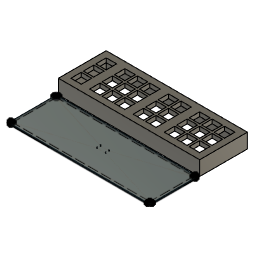
TIX Clock v4 (Autodesk Fusion 360 design; units mm, degrees)
Autodesk Fusion 360 part; units mm, degrees
note: some values were not read from the file. Set by a fixed rule: which face or edge a step refers to.
sketch "Sketch3" plane through (0, 0, 0) normal (0, 0, 1) x (1, 0, 0)
  line L0 (0, 0) -> (680, 0)
  line L1 (680, 0) -> (680, 230)
  line L2 (680, 230) -> (0, 230)
  line L3 (0, 230) -> (0, 0)
  dimension "d16" = 680
  dimension "d17" = 230
  constraint horizontal L0
  constraint vertical L1
  constraint horizontal L2
  constraint vertical L3
  constraint coincident L0.start L3.end
  measures "d16" distance of L0.start L0.end
  measures "d17" distance of L0.start L2.end
extrude "Extrude1" add sketch "Sketch3" along normal blind 70 makes body 1
sketch "Sketch4" plane through (0, 0, 70) normal (0, 0, 1) x (-1, 0, 0)
  line L0 (0, -230) -> (0, 0) construction
  line L1 (0, 0) -> (-680, 0)
  line L2 (-680, 0) -> (-680, -230)
  line L3 (-680, -230) -> (0, -230)
  line L4 (0, -200) -> (-680, -200)
  line L5 (0, -30) -> (-680, -30)
  line L6 (-30, -230) -> (-30, 0)
  line L7 (-650, -230) -> (-650, 0)
  line L8 (-80, -200) -> (-80, -30)
  line L9 (-120, -200) -> (-120, -30)
  line L10 (-170, -200) -> (-170, -30)
  line L11 (-180, -200) -> (-180, -30)
  line L12 (-230, -200) -> (-230, -30)
  line L13 (-30, -150) -> (-650, -150)
  line L14 (-30, -140) -> (-650, -140)
  line L15 (-30, -90) -> (-650, -90)
  line L16 (-30, -80) -> (-650, -80)
  line L17 (-30, -30) -> (-650, -30)
  line L18 (-240, -200) -> (-240, -30)
  line L19 (-290, -200) -> (-290, -30)
  line L20 (-330, -200) -> (-330, -30)
  line L21 (-380, -200) -> (-380, -30)
  line L22 (-390, -200) -> (-390, -30)
  line L23 (-440, -200) -> (-440, -30)
  line L24 (-480, -200) -> (-480, -30)
  line L25 (-530, -200) -> (-530, -30)
  line L26 (-540, -200) -> (-540, -30)
  line L27 (-590, -200) -> (-590, -30)
  line L28 (-600, -200) -> (-600, -30)
  line L29 (-650, -200) -> (-650, -30) construction
  dimension "d21" = 30
  dimension "d22" = 30
  dimension "d23" = 30
  dimension "d24" = 30
  dimension "d25" = 50
  dimension "d26" = 40
  dimension "d27" = 50
  dimension "d28" = 10
  dimension "d29" = 50
  dimension "d30" = 50
  dimension "d31" = 10
  dimension "d32" = 50
  dimension "d33" = 10
  dimension "d34" = 50
  dimension "d35" = 10
  dimension "d36" = 50
  dimension "d37" = 40
  dimension "d38" = 50
  dimension "d39" = 10
  dimension "d40" = 50
  dimension "d41" = 40
  dimension "d42" = 50
  dimension "d43" = 10
  dimension "d44" = 50
  dimension "d45" = 10
  dimension "d46" = 50
  constraint coincident L0 L4.start
  constraint perpendicular L0 L4
  constraint coincident L2 L4.end
  constraint coincident L0 L5.start
  constraint coincident L2 L5.end
  constraint perpendicular L2 L5
  constraint coincident L3 L6.start
  constraint coincident L1 L6.end
  constraint perpendicular L1 L6
  constraint coincident L3 L7.start
  constraint coincident L1 L7.end
  constraint perpendicular L1 L7
  constraint coincident L4 L8.start
  constraint coincident L5 L8.end
  constraint perpendicular L5 L8
  constraint coincident L4 L9.start
  constraint coincident L5 L9.end
  constraint perpendicular L5 L9
  constraint coincident L4 L10.start
  constraint coincident L5 L10.end
  constraint perpendicular L5 L10
  constraint coincident L4 L11.start
  constraint coincident L5 L11.end
  constraint perpendicular L5 L11
  constraint coincident L4 L12.start
  constraint coincident L5 L12.end
  constraint perpendicular L5 L12
  constraint coincident L7 L13.end
  constraint perpendicular L7 L13
  constraint coincident L6 L14.start
  constraint coincident L7 L14.end
  constraint perpendicular L7 L14
  constraint coincident L6 L15.start
  constraint coincident L7 L15.end
  constraint perpendicular L7 L15
  constraint coincident L6 L16.start
  constraint coincident L7 L16.end
  constraint perpendicular L7 L16
  constraint coincident L6 L17.start
  constraint coincident L7 L17.end
  constraint perpendicular L7 L17
  constraint coincident L4 L18.start
  constraint coincident L5 L18.end
  constraint coincident L4 L19.start
  constraint coincident L17 L19.end
  constraint coincident L4 L20.start
  constraint perpendicular L4 L20
  constraint coincident L4 L21.start
  constraint coincident L5 L21.end
  constraint coincident L4 L22.start
  constraint coincident L17 L22.end
  constraint coincident L4 L23.start
  constraint coincident L5 L23.end
  constraint perpendicular L5 L23
  constraint perpendicular L13 L24
  constraint coincident L4 L25.start
  constraint coincident L5 L25.end
  constraint coincident L4 L26.start
  constraint coincident L5 L26.end
  constraint coincident L4 L27.start
  constraint coincident L17 L27.end
  constraint coincident L4 L28.start
  constraint coincident L5 L28.end
  constraint coincident L4 L29.start
  constraint coincident L5 L17.end
  measures "d21" distance of L3 L4
  measures "d22" distance of L1 L5
  measures "d23" distance of L0 L6
  measures "d24" distance of L2 L7
  measures "d25" distance of L6 L8
  measures "d26" distance of L8 L9
  measures "d27" distance of L9 L10
  measures "d28" distance of L10 L11
  measures "d29" distance of L11 L12
  measures "d30" distance of L4 L13
  measures "d31" distance of L13 L14
  measures "d32" distance of L14 L15
  measures "d33" distance of L15 L16
  measures "d34" distance of L16 L17
  measures "d35" distance of L12 L18
  measures "d36" distance of L18 L19
  measures "d37" distance of L19 L20
  measures "d38" distance of L20 L21
  measures "d39" distance of L21 L22
  measures "d40" distance of L22 L23
  measures "d41" distance of L23 L24
  measures "d42" distance of L24 L25
  measures "d43" distance of L25 L26
  measures "d44" distance of L26 L27
  measures "d45" distance of L27 L28
  measures "d46" distance of L28 L29
extrude "Extrude2" cut sketch "Sketch4" against normal blind 170 contours L5 L6 L8 L16 L17 | L5 L7 L16 L17 L28 | L5 L9 L10 L16 L17 | L6 L8 L14 L15 | L5 L16 L17 L26 L27 | L7 L14 L15 L28 | L4 L7 L13 L28 | L5 L11 L12 L16 L17 | L9 L10 L14 L15 | L4 L6 L8 L13 | L5 L16 L17 L24 L25 | L14 L15 L26 L27 | L4 L13 L26 L27 | L5 L16 L17 L18 L19 | L11 L12 L14 L15 | L4 L9 L10 L13 | L5 L16 L17 L22 L23 | L14 L15 L24 L25 | L4 L13 L24 L25 | L5 L16 L17 L20 L21 | L14 L15 L18 L19 | L4 L11 L12 L13 | L14 L15 L22 L23 | L4 L13 L22 L23 | L14 L15 L20 L21 | L4 L13 L18 L19 | L4 L13 L20 L21 bodies 1
sketch "Sketch5" plane through (0, 0, 0) normal (0, 0, -1) x (1, 0, 0)
  line L0 (650, -30) -> (650, -80)
  line L1 (650, -80) -> (600, -80)
  line L2 (600, -80) -> (600, -30)
  line L3 (600, -30) -> (650, -30)
  line L4 (480, -150) -> (530, -150)
  line L5 (530, -150) -> (530, -200)
  line L6 (530, -200) -> (480, -200)
  line L7 (480, -200) -> (480, -150)
  line L8 (440, -90) -> (440, -140)
  line L9 (440, -140) -> (390, -140)
  line L10 (390, -140) -> (390, -90)
  line L11 (390, -90) -> (440, -90)
  line L12 (380, -30) -> (380, -80)
  line L13 (380, -80) -> (330, -80)
  line L14 (330, -80) -> (330, -30)
  line L15 (330, -30) -> (380, -30)
  line L16 (180, -200) -> (180, -150)
  line L17 (180, -150) -> (230, -150)
  line L18 (230, -150) -> (230, -200)
  line L19 (230, -200) -> (180, -200)
  line L20 (120, -140) -> (120, -90)
  line L21 (120, -90) -> (170, -90)
  line L22 (170, -90) -> (170, -140)
  line L23 (170, -140) -> (120, -140)
  line L24 (30, -30) -> (80, -30)
  line L25 (80, -30) -> (80, -80)
  line L26 (80, -80) -> (30, -80)
  line L27 (30, -80) -> (30, -30)
  line L28 (120, -200) -> (120, -150)
  line L29 (120, -150) -> (170, -150)
  line L30 (170, -150) -> (170, -200)
  line L31 (170, -200) -> (120, -200)
  line L32 (180, -140) -> (180, -90)
  line L33 (180, -90) -> (230, -90)
  line L34 (230, -90) -> (230, -140)
  line L35 (230, -140) -> (180, -140)
  line L36 (290, -30) -> (290, -80)
  line L37 (290, -80) -> (240, -80)
  line L38 (240, -80) -> (240, -30)
  line L39 (240, -30) -> (290, -30)
  line L40 (390, -150) -> (440, -150)
  line L41 (440, -150) -> (440, -200)
  line L42 (440, -200) -> (390, -200)
  line L43 (390, -200) -> (390, -150)
  line L44 (530, -90) -> (530, -140)
  line L45 (530, -140) -> (480, -140)
  line L46 (480, -140) -> (480, -90)
  line L47 (480, -90) -> (530, -90)
  line L48 (590, -30) -> (590, -80)
  line L49 (590, -80) -> (540, -80)
  line L50 (540, -80) -> (540, -30)
  line L51 (540, -30) -> (590, -30)
  line L52 (650, -90) -> (650, -140)
  line L53 (650, -140) -> (600, -140)
  line L54 (600, -140) -> (600, -90)
  line L55 (600, -90) -> (650, -90)
  line L56 (540, -150) -> (590, -150)
  line L57 (590, -150) -> (590, -200)
  line L58 (590, -200) -> (540, -200)
  line L59 (540, -200) -> (540, -150)
  line L60 (440, -30) -> (440, -80)
  line L61 (440, -80) -> (390, -80)
  line L62 (390, -80) -> (390, -30)
  line L63 (390, -30) -> (440, -30)
  line L64 (380, -90) -> (380, -140)
  line L65 (380, -140) -> (330, -140)
  line L66 (330, -140) -> (330, -90)
  line L67 (330, -90) -> (380, -90)
  line L68 (240, -150) -> (290, -150)
  line L69 (290, -150) -> (290, -200)
  line L70 (290, -200) -> (240, -200)
  line L71 (240, -200) -> (240, -150)
  line L72 (120, -80) -> (120, -30)
  line L73 (120, -30) -> (170, -30)
  line L74 (170, -30) -> (170, -80)
  line L75 (170, -80) -> (120, -80)
  line L76 (30, -90) -> (80, -90)
  line L77 (80, -90) -> (80, -140)
  line L78 (80, -140) -> (30, -140)
  line L79 (30, -140) -> (30, -90)
  line L80 (30, -150) -> (80, -150)
  line L81 (80, -150) -> (80, -200)
  line L82 (80, -200) -> (30, -200)
  line L83 (30, -200) -> (30, -150)
  line L84 (180, -80) -> (180, -30)
  line L85 (180, -30) -> (230, -30)
  line L86 (230, -30) -> (230, -80)
  line L87 (230, -80) -> (180, -80)
  line L88 (290, -90) -> (290, -140)
  line L89 (290, -140) -> (240, -140)
  line L90 (240, -140) -> (240, -90)
  line L91 (240, -90) -> (290, -90)
  line L92 (330, -150) -> (380, -150)
  line L93 (380, -150) -> (380, -200)
  line L94 (380, -200) -> (330, -200)
  line L95 (330, -200) -> (330, -150)
  line L96 (530, -30) -> (530, -80)
  line L97 (530, -80) -> (480, -80)
  line L98 (480, -80) -> (480, -30)
  line L99 (480, -30) -> (530, -30)
  line L100 (590, -90) -> (590, -140)
  line L101 (590, -140) -> (540, -140)
  line L102 (540, -140) -> (540, -90)
  line L103 (540, -90) -> (590, -90)
  line L104 (600, -200) -> (600, -150)
  line L105 (600, -150) -> (650, -150)
  line L106 (650, -150) -> (650, -200)
  line L107 (650, -200) -> (600, -200)
  line L108 (0, 0) -> (0, -230)
  line L109 (0, -230) -> (680, -230)
  line L110 (680, -230) -> (680, 0)
  line L111 (680, 0) -> (0, 0)
  line L112 (20, 0) -> (20, -230)
  line L113 (0, -20) -> (680, -20)
  line L114 (660, 0) -> (660, -230)
  line L115 (680, -210) -> (0, -210)
  dimension "d50" = 20
  dimension "d51" = 20
  dimension "d52" = 20
  dimension "d53" = 20
  constraint coincident L111 L112.start
  constraint coincident L109 L112.end
  constraint perpendicular L109 L112
  constraint coincident L108 L113.start
  constraint coincident L110 L113.end
  constraint perpendicular L110 L113
  constraint coincident L111 L114.start
  constraint coincident L109 L114.end
  constraint perpendicular L109 L114
  constraint coincident L110 L115.start
  constraint coincident L108 L115.end
  constraint perpendicular L108 L115
  measures "d50" distance of L108 L112
  measures "d51" distance of L111 L113
  measures "d52" distance of L110 L114
  measures "d53" distance of L109 L115
extrude "Extrude3" cut sketch "Sketch5" against normal blind 50 contours L112 L113 L114 L115 bodies 1
sketch "Sketch7" plane through (0, 0, 0) normal (0, 0, 1) x (1, 0, 0)
  line L0 (0, 0) -> (680, 0)
  line L1 (680, 0) -> (680, -230)
  line L2 (680, -230) -> (0, -230)
  line L3 (0, -230) -> (0, 0)
  dimension "d63" = 680
  dimension "d64" = 230
  constraint horizontal L0
  constraint vertical L1
  constraint horizontal L2
  constraint vertical L3
  constraint coincident L0.start L3.end
  measures "d63" distance of L1 L3
  measures "d64" distance of L0 L2
move_body "Move2" bodies 1 to x (1, 0, 0) y (0, 1, 0) z (0, 0, 1) at (0, 40, 0)
extrude "Extrude5" add sketch "Sketch7" along normal blind 5 separate body makes body 2
sketch "Sketch8" plane through (0, 0, 5) normal (0, 0, 1) x (-1, 0, 0)
  line L0 (0, 230) -> (-680, 230)
  line L1 (-680, 230) -> (-680, 0)
  line L2 (-680, 0) -> (0, 0)
  line L3 (0, 0) -> (0, 230)
  line L4 (-10, 0) -> (-10, 230) construction
  line L5 (0, 10) -> (-680, 10) construction
  line L6 (0, 220) -> (-680, 220) construction
  line L7 (-670, 230) -> (-670, 0) construction
  circle A0 centre (-10, 220) radius 5
  circle A1 centre (-10, 10) radius 5
  circle A2 centre (-670, 10) radius 5
  circle A3 centre (-670, 220) radius 5
  dimension "d71" = 10
  dimension "d72" = 10
  dimension "d73" = 10
  dimension "d74" = 10
  dimension "d75" = 10
  dimension "d76" = 10
  dimension "d77" = 10
  dimension "d78" = 10
  constraint coincident L2 L4.start
  constraint coincident L0 L4.end
  constraint perpendicular L0 L4
  constraint coincident L3 L5.start
  constraint coincident L1 L5.end
  constraint perpendicular L1 L5
  constraint coincident L3 L6.start
  constraint coincident L1 L6.end
  constraint perpendicular L1 L6
  constraint coincident L0 L7.start
  constraint coincident L2 L7.end
  constraint perpendicular L2 L7
  constraint coincident L6 A0.centre
  constraint coincident L4 A0.centre
  constraint coincident L4 A1.centre
  constraint coincident L5 A1.centre
  constraint coincident L5 A2.centre
  constraint coincident L7 A2.centre
  constraint coincident L6 A3.centre
  constraint coincident L7 A3.centre
  measures "d71" distance of L3 L4
  measures "d72" distance of L2 L5
  measures "d73" distance of L0 L6
  measures "d74" distance of L1 L7
  measures "d75" diameter of A0
  measures "d76" diameter of A1
  measures "d77" diameter of A2
  measures "d78" diameter of A3
extrude "Extrude6" cut sketch "Sketch8" against normal blind 5 contours A0 | A1 | A2 | A3 bodies 2
thread "Thread1" "ISO Metric profile 10.0 M10x1.5 6H" major diameter 10.198 minor diameter 8.526 pitch 1.5 angle 60 resizes the face on face at (5.0062, -9.7508, 1.6667) on face at (669.3783, -14.9612, 1.6667) on face at (669.3783, -224.9612, 1.6667) on bodies 2
sketch "Sketch9" plane through (0, 0, 0) normal (0, 0, -1) x (1, 0, 0)
  line L0 (660, -250) -> (20, -250)
  line L1 (20, -250) -> (20, -60)
  line L2 (20, -60) -> (660, -60)
  line L3 (660, -60) -> (660, -250)
  line L4 (0, -40) -> (0, -270)
  line L5 (0, -270) -> (680, -270)
  line L6 (680, -270) -> (680, -40)
  line L7 (680, -40) -> (0, -40)
  line L8 (670, -40) -> (670, -270) construction
  line L9 (680, -50) -> (0, -50) construction
  line L10 (680, -260) -> (0, -260) construction
  line L11 (10, -40) -> (10, -270) construction
  circle A0 centre (10, -50) radius 5
  circle A1 centre (670, -50) radius 5
  circle A2 centre (670, -260) radius 5
  circle A3 centre (10, -260) radius 5
  dimension "d81" = 10
  dimension "d82" = 10
  dimension "d83" = 10
  dimension "d84" = 10
  dimension "d85" = 10
  dimension "d86" = 10
  dimension "d87" = 10
  dimension "d88" = 10
  constraint coincident L7 L8.start
  constraint coincident L5 L8.end
  constraint perpendicular L5 L8
  constraint coincident L6 L9.start
  constraint coincident L4 L9.end
  constraint perpendicular L4 L9
  constraint coincident L6 L10.start
  constraint coincident L4 L10.end
  constraint perpendicular L4 L10
  constraint coincident L7 L11.start
  constraint perpendicular L10 L11
  constraint coincident L11 A0.centre
  constraint coincident L9 A0.centre
  constraint coincident L8 A1.centre
  constraint coincident L9 A1.centre
  constraint coincident L10 A2.centre
  constraint coincident L8 A2.centre
  constraint coincident L11 A3.centre
  constraint coincident L10 A3.centre
  measures "d81" distance of L6 L8
  measures "d82" distance of L7 L9
  measures "d83" distance of L5 L10
  measures "d84" distance of L4 L11
  measures "d85" diameter of A0
  measures "d86" diameter of A1
  measures "d87" diameter of A2
  measures "d88" diameter of A3
extrude "Extrude7" cut sketch "Sketch9" against normal blind 20 contours A0 | A1 | A2 | A3 bodies 1
thread "Thread2" "ISO Metric profile 10.0 M10x1.5 6H" major diameter 10.198 minor diameter 8.526 pitch 1.5 angle 60 resizes the face on face at (670.6217, 45.0388, 13.3333) on face at (670.6217, 255.0388, 13.3333) on face at (14.8454, 261.2338, 13.3333) on face at (14.9938, 50.2492, 13.3333) on bodies 1
sketch "Sketch10" plane through (0, 0, 5) normal (0, 0, 1) x (-1, 0, 0)
  circle A0 centre (-670, 10) radius 4.263
  circle A1 centre (-10, 220) radius 5
  circle A2 centre (-670, 220) radius 4.263
  circle A3 centre (-10, 10) radius 4.263
  line L0 (0, 230) -> (-680, 230)
  line L1 (-680, 230) -> (-680, 0)
  line L2 (-680, 0) -> (0, 0)
  line L3 (0, 0) -> (0, 230)
  line L4 (0, 106.5) -> (-680, 106.5) construction
  line L5 (0, 123.5) -> (-680, 123.5) construction
  line L6 (-680, 230) -> (0, 230)
  line L7 (-319.3, 0) -> (-319.3, 230) construction
  line L8 (0, 230) -> (0, 0) construction
  line L9 (-360.7, 0) -> (-360.7, 230) construction
  line L10 (-680, 0) -> (-680, 230) construction
  circle A4 centre (-319.3, 106.5) radius 1.9
  circle A5 centre (-319.3, 123.5) radius 1.9
  circle A6 centre (-360.7, 123.5) radius 1.9
  circle A7 centre (-360.7, 106.5) radius 1.9
  dimension "d92" = 106.5
  dimension "d95" = 106.5
  dimension "d96" = 319.3
  dimension "d97" = 319.3
  dimension "d101" = 3.8
  dimension "d103" = 3.8
  dimension "d104" = 3.8
  dimension "d105" = 3.8
  constraint coincident L3 L4.start
  constraint coincident L1 L4.end
  constraint perpendicular L1 L4
  constraint coincident L3 L5.start
  constraint coincident L1 L5.end
  constraint perpendicular L1 L5
  constraint coincident L2 L7.start
  constraint perpendicular L2 L7
  constraint coincident L2 L9.start
  constraint coincident L0 L9.end
  constraint perpendicular L0 L9
  constraint coincident L4 A4.centre
  constraint coincident L7 A4.centre
  constraint coincident L7 A5.centre
  constraint coincident L5 A5.centre
  constraint coincident L5 A6.centre
  constraint coincident L9 A6.centre
  constraint coincident L9 A7.centre
  constraint coincident L4 A7.centre
  measures "d92" distance of L2 L4
  measures "d95" distance of L5 L6
  measures "d96" distance of L7 L8
  measures "d97" distance of L9 L10
  measures "d101" diameter of A4
  measures "d103" diameter of A5
  measures "d104" diameter of A6
  measures "d105" diameter of A7
extrude "Extrude8" add sketch "Sketch10" along normal blind 4 contours A4 | A5 | A6 | A7 bodies 2
sketch "Sketch12" plane through (0, 0, 9) normal (0, 0, 1) x (-1, 0, 0)
  circle A0 centre (-360.7, 106.5) radius 1.9
  circle A1 centre (-360.7, 106.5) radius 1.05
  dimension "d108" = 2.1
  constraint concentric A0 A1
  measures "d108" diameter of A1
sketch "Sketch13" plane through (0, 0, 9) normal (0, 0, 1) x (-1, 0, 0)
  circle A0 centre (-360.7, 123.5) radius 1.9
  circle A1 centre (-360.7, 123.5) radius 1.05
  dimension "d109" = 2.1
  constraint concentric A0 A1
  measures "d109" diameter of A1
sketch "Sketch14" plane through (0, 0, 9) normal (0, 0, 1) x (-1, 0, 0)
  circle A0 centre (-319.3, 123.5) radius 1.9
  circle A1 centre (-319.3, 123.5) radius 1.05
  dimension "d110" = 2.1
  constraint concentric A0 A1
  measures "d110" diameter of A1
sketch "Sketch15" plane through (0, 0, 9) normal (0, 0, 1) x (-1, 0, 0)
  circle A0 centre (-319.3, 106.5) radius 1.9
  circle A1 centre (-319.3, 106.5) radius 1.05
  dimension "d111" = 2.1
  constraint concentric A0 A1
  measures "d111" diameter of A1
extrude "Extrude9" cut sketch "Sketch14" sketch "Sketch13" sketch "Sketch15" sketch "Sketch12" against normal blind 3 contours A1 of sketch 2 contours A1 of sketch 3 contours A1 of sketch 4 contours A1 bodies 2
thread "Thread3" "ISO Metric profile 2.0 M2x0.4 6H" major diameter 2.074 minor diameter 1.623 pitch 0.4 angle 60 resizes the face on face at (319.1177, -107.534, 7) on face at (319.1177, -124.534, 7) on face at (360.5177, -107.534, 7) on face at (360.5177, -124.534, 7) on bodies 2
move_body "MoveFace1" bodies 1 to x (1, 0, 0) y (0, 1, 0) z (0, 0, 1) at (0, -30, 0) on bodies 1
equation "RPP_totLen = 51 mm"
equation "RPP_totWidth = 21 mm"
equation "RPP_screwHoalDepthW = 2 mm" comment "Center"
equation "RPP_screwHoalDepthH = 4.8 mm" comment "Center"
equation "RPP_totThick = 1 mm"
equation "RPP_screwDiameterInner = 2.1 mm"
equation "LED_spacingUnit = 10 mm" comment "1 LED"
equation "LED_spacingSet = 40 mm" comment "Multiple units"
equation "LED_margin = 30 mm" comment "Outside set"
equation "d16 = BOX_length"
equation "d17 = BOX_width"
equation "BOX_height = 70 mm"
equation "d19 = BOX_height"
equation "d21 = LED_margin"
equation "d22 = LED_margin"
equation "d23 = LED_margin"
equation "d24 = LED_margin"
equation "d25 = LED_width"
equation "d26 = LED_spacingSet"
equation "d27 = LED_width"
equation "d28 = LED_spacingUnit"
equation "d29 = LED_width"
equation "d30 = LED_height"
equation "d31 = LED_spacingUnit"
equation "d32 = LED_height"
equation "d33 = LED_spacingUnit"
equation "d34 = LED_height"
equation "d35 = LED_spacingUnit"
equation "d36 = LED_width"
equation "d37 = LED_spacingSet"
equation "d38 = LED_width"
equation "d39 = LED_spacingUnit"
equation "d40 = LED_width"
equation "d41 = LED_spacingSet"
equation "d42 = LED_width"
equation "d43 = LED_spacingUnit"
equation "d44 = LED_width"
equation "d45 = LED_spacingUnit"
equation "d46 = LED_width"
equation "BOX_wallThicknes = 20 mm"
equation "d50 = BOX_wallThicknes"
equation "d51 = BOX_wallThicknes"
equation "d52 = BOX_wallThicknes"
equation "d53 = BOX_wallThicknes"
equation "d54 = -BOX_height + BOX_wallThicknes"
equation "d63 = BOX_length"
equation "d64 = BOX_width"
equation "BOX_bottomThickness = 5 mm"
equation "d69 = BOX_bottomThickness"
equation "d71 = BOX_wallThicknes / 2"
equation "d72 = BOX_wallThicknes / 2"
equation "d73 = BOX_wallThicknes / 2"
equation "d74 = BOX_wallThicknes / 2"
equation "d75 = BOX_wallThicknes / 2"
equation "d76 = BOX_wallThicknes / 2"
equation "d77 = BOX_wallThicknes / 2"
equation "d78 = BOX_wallThicknes / 2"
equation "d79 = -BOX_bottomThickness"
equation "d81 = BOX_wallThicknes / 2"
equation "d82 = BOX_wallThicknes / 2"
equation "d83 = BOX_wallThicknes / 2"
equation "d84 = BOX_wallThicknes / 2"
equation "d85 = BOX_wallThicknes / 2"
equation "d86 = BOX_wallThicknes / 2"
equation "d87 = BOX_wallThicknes / 2"
equation "d88 = BOX_wallThicknes / 2"
equation "BOX_screwHoal = 20 mm"
equation "d90 = -BOX_screwHoal"
equation "d92 = ( BOX_width / 2 ) - ( RPP_totWidth / 2 ) + RPP_screwFromEdgeW"
equation "BOX_length = ( LED_margin * 2 ) + ( LED_height * 9 ) + ( LED_spacingUnit * 5 ) + ( LED_spacingSet * 3 )"
equation "BOX_width = ( LED_margin * 2 ) + ( LED_width * 3 ) + ( LED_spacingUnit * 2 )"
equation "d95 = ( BOX_width / 2 ) - ( RPP_totWidth / 2 ) + RPP_screwFromEdgeW"
equation "d96 = ( BOX_length / 2 ) - ( RPP_totLen / 2 ) + RPP_screwFromEdgeL"
equation "d97 = ( BOX_length / 2 ) - ( RPP_totLen / 2 ) + RPP_screwFromEdgeL"
equation "RPP_screwFromEdgeL = 4.8 mm"
equation "RPP_screwFromEdgeW = 2 mm"
equation "d101 = RPP_screwDiameterOuter"
equation "RPP_screwDiameterOuter = 3.8 mm"
equation "d103 = RPP_screwDiameterOuter"
equation "d104 = RPP_screwDiameterOuter"
equation "d105 = RPP_screwDiameterOuter"
equation "d106 = RPP_totThick * 4"
equation "d108 = RPP_screwDiameterInner"
equation "d109 = RPP_screwDiameterInner"
equation "d110 = RPP_screwDiameterInner"
equation "d111 = RPP_screwDiameterInner"
equation "d112 = -RPP_totThick * 3"
equation "LED_width = 50 mm"
equation "LED_height = 50 mm"
